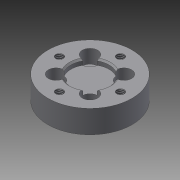
# Autodesk Inventor part: plate_cfs055ca501u
Saved by Autodesk Inventor 2013 (Build 170138000, 138)
## iProperties
Created: 2013-03-18
Part Number: plate_cfs055ca501u
Material: Generic
Document SubType Name: Modeling
Designer: Mahisorn
Density: 1 g/cm^3
Author: Mahisorn
Autodesk Inventor part; units mm, degrees
ref_plane "YZ Plane" through (0, 0, 0) normal (1, 0, 0) x (0, 1, 0)
ref_plane "XZ Plane" through (0, 0, 0) normal (0, 1, 0) x (-1, 0, 0)
ref_plane "XY Plane" through (0, 0, 0) normal (0, 0, 1) x (1, 0, 0)
sketch "Sketch1" plane through (0, 0, 0) normal (0, 0, 1) x (1, 0, 0)
  circle A0 centre (0, 0) radius 27.5
  dimension "d0" = 55
  constraints: 1 centre point, 1 coincident
  measures "d0" diameter of A0
extrude "Extrusion1" add sketch "Sketch1" along normal blind 15
sketch "Sketch2" plane through (0, 0, 15) normal (0, 0, 1) x (1, 0, 0)
  circle A0 centre (0, 0) radius 27.5 projected
  circle A1 centre (0, 0) radius 12.5
  point P0 (15.75, 0)
  point P1 (20, 0)
  point P2 (11.1369, 11.1369)
  point P3 (0, 15.75)
  point P4 (-11.1369, 11.1369)
  point P5 (-15.75, 0)
  point P6 (-11.1369, -11.1369)
  point P7 (0, -15.75)
  point P8 (11.1369, -11.1369)
  point P9 (14.1421, 14.1421)
  point P10 (0, 20)
  point P11 (-14.1421, 14.1421)
  point P12 (-20, 0)
  point P13 (-14.1421, -14.1421)
  point P14 (0, -20)
  point P15 (14.1421, -14.1421)
  dimension "d3" = 15.75
  dimension "d4" = 20
  dimension "d7" = 360
  dimension "d11" = 360
  dimension "d13" = 25
  constraints: 1 centre point, 1 coincident, 18 other
  measures "d3" distance of A0.centre point (15.75, 0)
  measures "d4" distance of A0.centre point (20, 0)
  measures "d13" diameter of A1
extrude "Extrusion2" cut sketch "Sketch2" against normal blind 3.5 contours A1
hole "Hole1" at (-11.1369, 11.1369, 15) at (-11.1369, -11.1369, 15) at (11.1369, 11.1369, 15) at (11.1369, -11.1369, 15) direction (0, 0, -1) diameter 5.5 end through all counterbore diameter 10 counterbore depth 9 clearance for "Socket Head Cap Screw ISO 4762" size "M5" standard "ISO"
hole "Hole2" at (0, 20, 15) at (-20, 0, 15) at (0, -20, 15) at (20, 0, 15) direction (0, 0, -1) diameter 4.917 depth 10 tip angle 118 thread size "M6x1" class "6H" standard "ANSI Metric M Profile"
sketch "Sketch3" plane through (0, 0, 0) normal (0, 0, -1) x (-1, 0, 0)
  circle A0 centre (0, 0) radius 27.5 projected
  circle A1 centre (0, 0) radius 10
  point P0 (-15.75, 0)
  dimension "d31" = 15.75
  dimension "d32" = 20
  constraints: 1 centre point, 1 coincident
  measures "d31" distance of point (-15.75, 0) A0.centre
  measures "d32" diameter of A1
hole "Hole3" at (15.75, 0, 0) direction (0, 0, 1) diameter 3 depth 4 tip angle 118
extrude "Extrusion3" add sketch "Sketch3" along normal blind 3 contours A1
chamfer "Chamfer1" distance 1 angle 45 1 edges at (10, 0, -3)
chamfer "Chamfer2" distance 1 angle 45 4 edges at (12.5, 0, 15) (0, 12.5, 15) (0, -12.5, 15) (-12.5, 0, 15)
body "Solid1"
